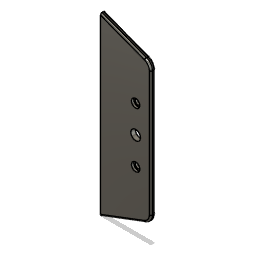
ZED mount Tassen (Autodesk Fusion 360 archive; units mm, degrees)
design "ZedCameraMountV2"
Autodesk Fusion 360 part; units mm, degrees
sketch "Sketch1" plane through (0, 0, 0) normal (0, 0, 1) x (1, 0, 0)
  line L0 (0, 0) -> (0, 57.5)
  line L1 (0, 57.5) -> (29.1254, 46.4677)
  line L2 (33, 40.8567) -> (33, -40.8567)
  line L3 (29.1254, -46.4677) -> (0, -57.5)
  line L4 (0, -57.5) -> (0, 0)
  arc A0 (29.1254, -46.4677) -> (33, -40.8567) centre (27, -40.8567) ccw
  arc A1 (33, 40.8567) -> (29.1254, 46.4677) centre (27, 40.8567) ccw
  point P0 (33, 45)
  point P1 (33, -45)
  dimension "d1" = 90
  dimension "d2" = 115
  dimension "d3" = 33
  dimension "d4" = 6
  constraint coincident L0.start L4.end
  constraint vertical L0
  constraint parallel L0 L2
  constraint parallel L0 L4
  constraint equal L0 L4
  constraint coincident P1 L2
  constraint coincident P1 L3
  constraint tangent L2 A0
  constraint tangent L3 A0
  constraint coincident P0 L1
  constraint coincident P0 L2
  constraint tangent L1 A1
  constraint tangent L2 A1
  constraint equal A0 A1
  measures "d1" distance of P0 P1
  measures "d2" distance of L0.end L3.end
  measures "d3" distance of L0 L2
  measures "d4" radius of A0
extrude "Extrude1" add sketch "Sketch1" along normal blind 3
sketch "Sketch2" plane through (0, 0, 3) normal (0, 0, 1) x (1, 0, 0)
  arc A0 (29.1254, -46.4677) -> (33, -40.8567) centre (27, -40.8567) ccw
  line L0 (33, -40.8567) -> (33, 40.8567)
  arc A1 (33, 40.8567) -> (29.1254, 46.4677) centre (27, 40.8567) ccw
  line L1 (29.1254, 46.4677) -> (0, 57.5)
  line L2 (0, 57.5) -> (0, -57.5)
  line L3 (0, -57.5) -> (29.1254, -46.4677)
  line L4 (23, -48.7879) -> (23, 48.7879) construction
  circle A2 centre (23, 0) radius 3.2
  circle A3 centre (23, 18) radius 1.5
  circle A4 centre (23, -18) radius 1.5
  dimension "d7" = 10
  dimension "d8" = 6.4
  dimension "d9" = 3
  dimension "d11" = 36
  dimension "d12" = 18
  constraint coincident L3 L4.start
  constraint coincident L1 L4.end
  constraint vertical L4
  constraint midpoint L4 A2.centre
  constraint coincident L4 A3.centre
  constraint coincident L4 A4.centre
  constraint equal A3 A4
  measures "d7" distance of L0 L4
  measures "d8" diameter of A2
  measures "d9" diameter of A4
  measures "d11" distance of A3.centre A4.centre
  measures "d12" distance of A2.centre A4.centre
hole "Hole1" at (23, 0, 3) direction (0, 0, -1) diameter 6.4 end up to surface (3 mm away)
hole "Hole2" at (23, -18, 3) at (23, 18, 3) direction (0, 0, -1) diameter 3.5 depth 3 tip angle 118 counterbore diameter 5.5 counterbore depth 1.5
fillet "Fillet1" radius 1 10 edges at (14.5627, -51.9838, 3) (31.9372, -44.2661, 3) (33, 0, 3) (31.9372, 44.2661, 3) (14.5627, 51.9838, 3) (14.5627, 51.9838, 0) (31.9372, 44.2661, 0) (33, 0, 0) (31.9372, -44.2661, 0) (14.5627, -51.9838, 0)
equation "d8 = ( 25.6 / 4 ) * 1 mm"
